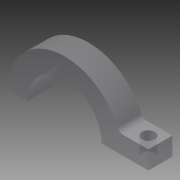
# Autodesk Inventor part: GE-13039
Saved by Autodesk Inventor 2013 (Build 170138000, 138)
## iProperties
Created: 2013-01-06
Part Number: GE-13039
Material: Polycarbonate, Clear
Document SubType Name: Modeling
Designer: Phillip
Density: 1 g/cm^3
Author: Phillip
Autodesk Inventor part; units mm, degrees
ref_plane "YZ Plane" through (0, 0, 0) normal (1, 0, 0) x (0, 1, 0)
ref_plane "XZ Plane" through (0, 0, 0) normal (0, 1, 0) x (-1, 0, 0)
ref_plane "XY Plane" through (0, 0, 0) normal (0, 0, 1) x (1, 0, 0)
sketch "Sketch1" plane through (0, 0, 0) normal (0, 0, 1) x (1, 0, 0)
  arc A0 (19.685, 0) -> (-19.685, 0) centre (0, 0) ccw
  arc A1 (28.6435, 9.652) -> (-30.226, 0) centre (0, 0) ccw
  line L0 (44.45, 0) -> (44.45, 9.652)
  line L1 (44.45, 9.652) -> (28.6435, 9.652)
  line L2 (-30.226, 0) -> (-19.685, 0)
  line L3 (19.685, 0) -> (44.45, 0)
  dimension "d0" = 39.37
  dimension "d1" = 60.452
  dimension "d2" = 44.45
  dimension "d15" = 9.652
  constraints: 8 end point, 4 point on circle, 2 centre point, 2 coincident, 2 horizontal, 2 parallel, 1 vertical
  measures "d0" diameter of A0
  measures "d1" diameter of A1
  measures "d2" distance from line of L0 A0.centre
  measures "d15" distance between parallel lines of L1 L3
extrude "Extrusion1" add sketch "Sketch1" against normal blind 12.7
fillet "Fillet1" radius 3.175 1 edges at (28.6435, 9.652, -6.35)
sketch "Sketch2" plane through (44.45, 9.652, 0) normal (0, 1, 0) x (1, 0, 0)
  line L0 (0, 0) -> (0, 12.7) projected
  line L1 (-13.6102, 12.7) -> (0, 12.7) projected
  point P0 (-44.45, 0)
  point P1 (-6.35, 6.35)
  dimension "d6" = 6.35
  dimension "d7" = 6.35
  measures "d6" distance from line of point (-6.35, 6.35) L0
  measures "d7" distance from line of L1 point (-6.35, 6.35)
hole "Hole1" at (38.1, 9.652, -6.35) direction (0, -1, 0) diameter 6.858 end through all
equation "\"d7\" = d6"
body "Solid1"
